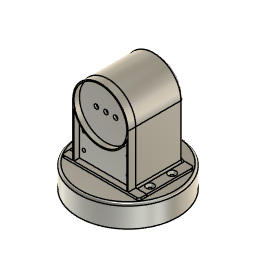
TRARM02_Link1 (Autodesk Fusion 360 design; units mm, degrees)
Autodesk Fusion 360 part; units mm, degrees
sketch "스케치1" plane through (0, 0, 0) normal (0, 0, 1) x (1, 0, 0) in component "TRARM02_Link1A_R90x20 v1"
  circle A0 centre (0, 0) radius 45
  dimension "d1" = 90
  constraint coincident A0.centre origin
  measures "d1" diameter of A0
extrude "돌출1" add sketch "스케치1" along normal blind 2 makes body 1 in component "TRARM02_Link1A_R90x20 v1"
sketch "스케치2" plane through (0, 0, 2) normal (0, 0, 1) x (-1, 0, 0) in component "TRARM02_Link1A_R90x20 v1"
  circle A0 centre (0, 0) radius 45
  circle A1 centre (0, 0) radius 43
  dimension "d4" = 86
  dimension "d5" = 90
  constraint coincident A0.centre A1.centre
  measures "d4" diameter of A1
  measures "d5" diameter of A0
extrude "돌출2" add sketch "스케치2" along normal blind 18 bodies 1 in component "TRARM02_Link1A_R90x20 v1"
fillet "필렛1" radius 2 1 edges at (-41.9547, -16.2727, 0) on bodies 1 in component "TRARM02_Link1A_R90x20 v1"
sketch "스케치4" plane through (0, 0, 2) normal (0, 0, 1) x (-1, 0, 0) in component "TRARM02_Link1A_R90x20 v1"
  circle A0 centre (0, 0) radius 43
  line L0 (-30, -13) -> (-40.9878, -13)
  line L1 (-30, -7) -> (-42.4264, -7)
  line L2 (-30, 7) -> (-42.4264, 7)
  line L3 (-30, 13) -> (-40.9878, 13)
  line L4 (30, -13) -> (40.9878, -13)
  line L5 (30, -7) -> (42.4264, -7)
  line L6 (30, 7) -> (42.4264, 7)
  line L7 (30, 13) -> (40.9878, 13)
  arc A1 (30, 13) -> (30, 7) centre (30, 10) ccw
  arc A2 (30, -7) -> (30, -13) centre (30, -10) ccw
  arc A3 (-30, -13) -> (-30, -7) centre (-30, -10) ccw
  arc A4 (-30, 7) -> (-30, 13) centre (-30, 10) ccw
  dimension "d32" = 6
  dimension "d33" = 60
  dimension "d34" = 20
  dimension "d35" = 10
  dimension "d36" = 30
  dimension "d46" = 6
  dimension "d47" = 6
  constraint equal A2 A3
  constraint equal A1 A2
  constraint equal A1 A4
  constraint horizontal A2.centre A3.centre
  constraint horizontal A1.centre A4.centre
  constraint vertical A2.centre A1.centre
  constraint vertical A3.centre A4.centre
  constraint coincident A0 L0.end
  constraint coincident A0 L1.end
  constraint horizontal L0
  constraint horizontal L1
  constraint coincident A0 L2.end
  constraint coincident A0 L3.end
  constraint horizontal L2
  constraint horizontal L3
  constraint coincident A0 L4.end
  constraint coincident A0 L5.end
  constraint horizontal L4
  constraint horizontal L5
  constraint coincident A0 L6.end
  constraint coincident A0 L7.end
  constraint horizontal L6
  constraint horizontal L7
  constraint vertical L6.start L7.start
  constraint vertical L5.start L7.start
  constraint vertical L4.start L5.start
  constraint vertical L0.start L1.start
  constraint vertical L1.start L2.start
  constraint vertical L2.start L3.start
  measures "d32" diameter of A3
  measures "d33" distance of A2.centre A3.centre
  measures "d34" distance of A2.centre A1.centre
  measures "d35" vertical distance of A0.centre A1.centre
  measures "d36" horizontal distance of A0.centre A2.centre
  measures "d46" distance of L4 L5
  measures "d47" distance of L0 L1
extrude "돌출7" add sketch "스케치4" along normal blind 5 contours A0 L6 L7 A1 | A0 L4 L5 A2 | A0 L2 L3 A4 | A0 L0 L1 A3 bodies 1 in component "TRARM02_Link1A_R90x20 v1"
sketch "스케치7" plane through (0, 0, 0) normal (0, 0, -1) x (1, 0, 0) in component "TRARM02_Link1A_R90x20 v1"
  arc A0 (-30, -13) -> (-30, -7) centre (-30, -10) ccw construction
  arc A1 (-30, 7) -> (-30, 13) centre (-30, 10) ccw construction
  arc A2 (30, 13) -> (30, 7) centre (30, 10) ccw construction
  arc A3 (30, -7) -> (30, -13) centre (30, -10) ccw construction
  circle A4 centre (-30, 10) radius 1.45
  circle A5 centre (-30, -10) radius 1.45
  circle A6 centre (30, -10) radius 1.45
  circle A7 centre (30, 10) radius 1.45
  dimension "d42" = 2.9
  constraint concentric A1 A4
  constraint concentric A0 A5
  constraint concentric A3 A6
  constraint concentric A2 A7
  constraint equal A6 A7
  constraint equal A5 A6
  constraint equal A4 A5
  measures "d42" diameter of A7
extrude "돌출8" cut sketch "스케치7" against normal blind 5 bodies 1 in component "TRARM02_Link1A_R90x20 v1"
fillet "필렛2" radius 1 12 edges at (-35.4939, -13, 7) (-27, -10, 7) (-36.2132, -7, 7) (-36.2132, 7, 7) (-27, 10, 7) (-35.4939, 13, 7) (35.4939, 13, 7) (27, 10, 7) (36.2132, 7, 7) (36.2132, -7, 7) (27, -10, 7) (35.4939, -13, 7) on bodies 1 in component "TRARM02_Link1A_R90x20 v1"
sketch "스케치9" plane through (0, 0, 2) normal (0, 0, 1) x (-1, 0, 0) in component "TRARM02_Link1A_R90x20 v1"
  circle A0 centre (0, 0) radius 15
  dimension "d50" = 30
  constraint coincident A0.centre origin
  measures "d50" diameter of A0
extrude "돌출9" add sketch "스케치9" along normal blind 1 bodies 1 in component "TRARM02_Link1A_R90x20 v1"
sketch "스케치10" plane through (0, 0, 3) normal (0, 0, 1) x (-1, 0, 0) in component "TRARM02_Link1A_R90x20 v1"
  circle A0 centre (0, 0) radius 2
  circle A1 centre (-8.7, 0) radius 2
  circle A2 centre (8.7, 0) radius 2
  dimension "d53" = 8.7
  dimension "d54" = 8.7
  dimension "d55" = 4
  constraint coincident A0.centre origin
  constraint equal A0 A2
  constraint equal A1 A2
  constraint horizontal A0.centre A1.centre
  constraint horizontal A0.centre A2.centre
  measures "d53" distance of A0.centre A1.centre
  measures "d54" distance of A0.centre A2.centre
  measures "d55" diameter of A1
extrude "돌출10" cut sketch "스케치10" against normal blind 3 bodies 1 in component "TRARM02_Link1A_R90x20 v1"
sketch "스케치11" plane through (0, 0, 0) normal (0, 0, -1) x (1, 0, 0) in component "TRARM02_Link1A_R90x20 v1"
  line L0 (21, 5) -> (21, -5)
  line L1 (16, -5) -> (16, 5)
  line L2 (-16, 5) -> (-16, -5)
  line L3 (-21, -5) -> (-21, 5)
  arc A0 (-16, 5) -> (-21, 5) centre (-18.5, 5) ccw
  arc A1 (-21, -5) -> (-16, -5) centre (-18.5, -5) ccw
  arc A2 (16, -5) -> (21, -5) centre (18.5, -5) ccw
  arc A3 (21, 5) -> (16, 5) centre (18.5, 5) ccw
  dimension "d58" = 5
  dimension "d60" = 10
  dimension "d61" = 16
  dimension "d62" = 5
  dimension "d63" = 16
  dimension "d64" = 2.5
  dimension "d65" = 5
  constraint vertical L0
  constraint vertical L1
  constraint vertical L2
  constraint vertical L3
  constraint equal L0 L2
  constraint horizontal L1.start L2.end
  constraint equal A2 A3
  constraint equal A0 A1
  constraint equal A0 A2
  constraint horizontal L3.end L2.start
  constraint horizontal L1.end L3.end
  constraint horizontal L1.end L0.start
  constraint equal L2 L3
  measures "d58" distance of L0.end L1.start
  measures "d60" distance of L0.start L0.end
  measures "d61" horizontal distance of origin L1.start
  measures "d62" vertical distance of origin L1.start
  measures "d63" horizontal distance of origin L2.end
  measures "d64" radius of A2
  measures "d65" distance of L2 L3
extrude "돌출11" cut sketch "스케치11" against normal blind 2 bodies 1 in component "TRARM02_Link1A_R90x20 v1"
move_body "이동1" bodies 1 to x (1, 0, 0) y (0, -1, 0) z (0, 0, -1) at (0, 0, 0) in component "TRARM02_Link1A_R90x20 v1"
move_body "이동2" bodies 1 to x (1, 0, 0) y (0, 1, 0) z (0, 0, 1) at (0, 0, 20) in component "TRARM02_Link1A_R90x20 v1"
move_body "이동3" bodies 1 to x (0, 1, 0) y (-1, 0, 0) z (0, 0, 1) at (0, 0, 0) in component "TRARM02_Link1A_R90x20 v1"
move_body "이동4" bodies 1 to x (0, 1, 0) y (-1, 0, 0) z (0, 0, 1) at (0, 0, 0) in component "TRARM02_Link1A_R90x20 v1"
sketch "스케치1 (2)" plane through (0, 0, 0) normal (0, 0, 1) x (1, 0, 0) in component "TRARM02_Link1B_50x50x43 v1"
  line L0 (25, 50) -> (25, 2)
  line L1 (-25, 50) -> (-25, 2)
  arc A0 (25, 50) -> (-25, 50) centre (0, 50) ccw
  line L2 (-35, 0) -> (-35, 2)
  line L3 (-35, 2) -> (-25, 2)
  line L4 (35, 0) -> (35, 2)
  line L5 (35, 2) -> (25, 2)
  line L6 (-35, 0) -> (35, 0)
  dimension "d222" = 25
  dimension "d223" = 50
  dimension "d224" = 2
  dimension "d225" = 10
  constraint vertical origin A0.centre
  constraint vertical L0
  constraint tangent L1 A0
  constraint parallel L0 L1
  constraint vertical L2
  constraint horizontal L3
  constraint vertical L4
  constraint horizontal L5
  constraint perpendicular L2 L6
  constraint equal L2 L4
  constraint equal L3 L5
  constraint tangent L0 A0
  constraint coincident origin L6
  measures "d222" radius of A0
  measures "d223" distance of origin A0.centre
  measures "d224" distance of L4.start L4.end
  measures "d225" distance of L4.end L0.end
extrude "돌출1'" add sketch "스케치1 (2)" along normal blind 43 separate body makes body 2 in component "TRARM02_Link1B_50x50x43 v1"
sketch "스케치27" plane through (0, 0, 43) normal (0, 0, 1) x (-1, 0, 0) in component "TRARM02_Link1B_50x50x43 v1"
  line L0 (35, 0) -> (-35, 0)
  line L1 (24, -2) -> (-24, -2)
  line L2 (-20, -22) -> (-24, -22)
  line L3 (-20, -28) -> (-24, -28)
  line L4 (-20, -13) -> (-24, -13)
  line L5 (-20, -7) -> (-24, -7)
  line L6 (20, -13) -> (24, -13)
  line L7 (20, -7) -> (24, -7)
  line L8 (20, -22) -> (24, -22)
  line L9 (20, -28) -> (24, -28)
  arc A0 (20.0014, -22) -> (20, -28) centre (20, -25) ccw
  line L10 (24, -50) -> (24, -28)
  line L11 (24, -22) -> (24, -13)
  line L12 (24, -7) -> (24, -2)
  arc A1 (20, -7) -> (20, -13) centre (20, -10) ccw
  arc A2 (-20, -13) -> (-20, -7) centre (-20, -10) ccw
  line L13 (-24, -7) -> (-24, -2)
  arc A3 (-20, -28) -> (-20.0014, -22) centre (-20, -25) ccw
  line L14 (-24, -50) -> (-24, -28)
  line L15 (-24, -22) -> (-24, -13)
  line L16 (-3, -70) -> (-3, -73.8118)
  line L17 (3, -70) -> (3, -73.8118)
  arc A4 (3, -70) -> (-3, -70) centre (0, -70) ccw
  arc A5 (-24, -50) -> (-3, -73.8118) centre (0, -50) ccw
  arc A6 (3, -73.8118) -> (24, -50) centre (0, -50) ccw
  dimension "d246" = 48
  dimension "d247" = 50
  dimension "d248" = 2
  dimension "d251" = 6
  dimension "d252" = 20
  dimension "d253" = 25
  dimension "d254" = 15
  dimension "d255" = 20
  dimension "d279" = 6
  dimension "d280" = 20
  constraint parallel L0 L1
  constraint coincident L1 L13.end
  constraint vertical L10
  constraint vertical L14
  constraint coincident L1.end L13.end
  constraint tangent L14 A5
  constraint tangent L10 A5
  constraint vertical origin A5.centre
  constraint equal A0 A1
  constraint equal A0 A3
  constraint equal A2 A3
  constraint horizontal A2.centre A1.centre
  constraint horizontal A0.centre A3.centre
  constraint vertical A3.centre A2.centre
  constraint vertical A0.centre A1.centre
  constraint coincident L2.start A3
  constraint coincident L2.end L14
  constraint perpendicular L2 L14
  constraint perpendicular L3 L14
  constraint perpendicular L4 L14
  constraint coincident L5.end L14
  constraint perpendicular L5 L14
  constraint coincident L6.end L10
  constraint perpendicular L6 L10
  constraint coincident L7.end L10
  constraint perpendicular L7 L10
  constraint coincident L8.start A0
  constraint coincident L8.end L10
  constraint perpendicular L8 L10
  constraint perpendicular L9 L10
  constraint coincident L8 A0.start
  constraint collinear L10 L11
  constraint collinear L11 L12
  constraint collinear L13 L14
  constraint coincident L2 A3.end
  constraint collinear L14 L15
  constraint equal L2 L3
  constraint equal L2 L4
  constraint equal L4 L5
  constraint equal L5 L7
  constraint equal L6 L7
  constraint equal L6 L8
  constraint equal L8 L9
  constraint vertical A5.centre A4.centre
  constraint vertical L16
  constraint coincident L17.end A5
  constraint parallel L16 L17
  constraint concentric A5 A6
  constraint horizontal A4.centre L17.start
  constraint horizontal L16.start L17.start
  measures "d246" diameter of A5
  measures "d247" distance of origin A5.centre
  measures "d248" distance of origin L1
  measures "d251" diameter of A3
  measures "d252" horizontal distance of A5.centre A3.centre
  measures "d253" vertical distance of A5.centre A3.centre
  measures "d254" vertical distance of A3.centre A2.centre
  measures "d255" horizontal distance of A5.centre A0.centre
  measures "d279" diameter of A4
  measures "d280" distance of A5.centre A4.centre
extrude "돌출32" cut sketch "스케치27" against normal blind 41 bodies 2 in component "TRARM02_Link1B_50x50x43 v1"
sketch "스케치28" plane through (0, 0, 43) normal (0, 0, 1) x (-1, 0, 0) in component "TRARM02_Link1B_50x50x43 v1"
  circle A0 centre (-20, -25) radius 1.45
  circle A1 centre (-20, -10) radius 1.45
  circle A2 centre (20, -10) radius 1.45
  circle A3 centre (20, -25) radius 1.45
  arc A4 (-20, -28) -> (-20.0014, -22) centre (-20, -25) ccw
  arc A5 (-20, -13) -> (-20, -7) centre (-20, -10) ccw
  arc A6 (20, -7) -> (20, -13) centre (20, -10) ccw
  arc A7 (20.0014, -22) -> (20, -28) centre (20, -25) ccw
  circle A8 centre (0, -70) radius 1.45
  arc A9 (3, -70) -> (-3, -70) centre (0, -70) ccw
  dimension "d258" = 2.9
  constraint equal A0 A3
  constraint equal A0 A1
  constraint concentric A0 A4
  constraint concentric A1 A5
  constraint concentric A2 A6
  constraint concentric A3 A7
  constraint equal A0 A2
  constraint concentric A8 A9
  constraint equal A0 A8
  measures "d258" diameter of A0
extrude "돌출33" cut sketch "스케치28" against normal blind 5 bodies 2 in component "TRARM02_Link1B_50x50x43 v1"
fillet "필렛6" radius 2 3 edges at (-25, 26, 0) (0, 75, 0) (25, 26, 0) on bodies 2 in component "TRARM02_Link1B_50x50x43 v1"
fillet "필렛6" radius 2 2 edges at (35, 1, 0) (-35, 1, 0) on bodies 2 in component "TRARM02_Link1B_50x50x43 v1"
sketch "스케치29" plane through (0, 2, 0) normal (0, 1, 0) x (-1, 0, 0) in component "TRARM02_Link1B_50x50x43 v1"
  circle A0 centre (30, 15) radius 1.5
  circle A1 centre (30, 35) radius 1.5
  line L0 (25, 43) -> (35, 43)
  circle A2 centre (-30, 15) radius 1.5
  circle A3 centre (-30, 35) radius 1.5
  point P0 (-35, 43)
  dimension "d265" = 3
  dimension "d266" = 5
  dimension "d268" = 15
  dimension "d269" = 20
  dimension "d281" = 60
  constraint equal A2 A3
  constraint equal A0 A2
  constraint equal A0 A1
  constraint vertical A2.centre A3.centre
  constraint vertical A0.centre A1.centre
  constraint horizontal A0.centre A2.centre
  constraint horizontal A1.centre A3.centre
  measures "d265" diameter of A2
  measures "d266" horizontal distance of A1.centre L0.end
  measures "d268" vertical distance of origin A2.centre
  measures "d269" distance of A2.centre A3.centre
  measures "d281" distance of A1.centre A3.centre
extrude "돌출34" cut sketch "스케치29" against normal blind 2 bodies 2 in component "TRARM02_Link1B_50x50x43 v1"
chamfer "챔퍼6" distance 2 angle 45 4 edges at (31.3985, 2, 15.5424) (31.3985, 2, 35.5424) (-28.6015, 2, 35.5424) (-28.6015, 2, 15.5424) on bodies 2 in component "TRARM02_Link1B_50x50x43 v1"
fillet "필렛7" radius 1.4 4 edges at (24.4142, 2, 0.5858) (25, 2, 22.5) (-24.4142, 2, 0.5858) (-25, 2, 22.5) on bodies 2 in component "TRARM02_Link1B_50x50x43 v1"
sketch "스케치30" plane through (0, 0, 0) normal (0, -1, 0) x (1, 0, 0) in component "TRARM02_Link1B_50x50x43 v1"
  circle A0 centre (0, 25) radius 15
  line L0 (21, 30) -> (21, 20)
  line L1 (16, 20) -> (16, 30)
  arc A1 (21, 30) -> (16, 30) centre (18.5, 30) ccw
  arc A2 (16, 20) -> (21, 20) centre (18.5, 20) ccw
  line L2 (-16, 30) -> (-16, 20)
  line L3 (-21, 20) -> (-21, 30)
  arc A3 (-16, 30) -> (-21, 30) centre (-18.5, 30) ccw
  arc A4 (-21, 20) -> (-16, 20) centre (-18.5, 20) ccw
  dimension "d275" = 30
  dimension "d276" = 25
  dimension "d282" = 10
  dimension "d283" = 5
  dimension "d284" = 16
  dimension "d285" = 20
  dimension "d286" = 2.5
  dimension "d287" = 16
  dimension "d288" = 5
  dimension "d289" = 10
  dimension "d290" = 20
  dimension "d291" = 2.5
  constraint vertical origin A0.centre
  constraint vertical L0
  constraint vertical L1
  constraint equal A1 A2
  constraint equal L0 L1
  constraint horizontal L1.end L0.start
  constraint vertical L2
  constraint vertical L3
  constraint equal A3 A4
  constraint equal L2 L3
  constraint horizontal L2.end A4.centre
  constraint horizontal L2.end L3.start
  measures "d275" diameter of A0
  measures "d276" distance of origin A0.centre
  measures "d282" distance of L0.start L0.end
  measures "d283" distance of L0.end L1.start
  measures "d284" horizontal distance of origin L1.start
  measures "d285" vertical distance of origin L1.start
  measures "d286" radius of A2
  measures "d287" horizontal distance of origin L2.end
  measures "d288" distance of L3.end L2.start
  measures "d289" distance of L3.end L3.start
  measures "d290" vertical distance of origin L2.end
  measures "d291" radius of A4
extrude "돌출35" cut sketch "스케치30" against normal blind 2 bodies 2 in component "TRARM02_Link1B_50x50x43 v1"
sketch "스케치1 (3)" plane through (0, 0, 0) normal (0, 0, 1) x (1, 0, 0) in component "TRARM02_Link1C_50x50x7 v1"
  line L0 (25, 50) -> (25, 2)
  line L1 (-25, 50) -> (-25, 2)
  arc A0 (25, 50) -> (-25, 50) centre (0, 50) ccw
  line L2 (-35, 0) -> (-35, 2)
  line L3 (-35, 2) -> (-25, 2)
  line L4 (35, 0) -> (35, 2)
  line L5 (35, 2) -> (25, 2)
  line L6 (-35, 0) -> (35, 0)
  dimension "d222_1" = 25
  dimension "d223_1" = 50
  dimension "d224_1" = 2
  dimension "d225_1" = 10
  constraint vertical origin A0.centre
  constraint vertical L0
  constraint tangent L1 A0
  constraint parallel L0 L1
  constraint vertical L2
  constraint horizontal L3
  constraint vertical L4
  constraint horizontal L5
  constraint perpendicular L2 L6
  constraint equal L2 L4
  constraint equal L3 L5
  constraint tangent L0 A0
  constraint coincident origin L6
  measures "d222_1" radius of A0
  measures "d223_1" distance of origin A0.centre
  measures "d224_1" distance of L4.start L4.end
  measures "d225_1" distance of L4.end L0.end
extrude "돌출1''" add sketch "스케치1 (3)" along normal blind 7 separate body makes body 3 in component "TRARM02_Link1C_50x50x7 v1"
sketch "스케치24" plane through (0, 0, 7) normal (0, 0, 1) x (-1, 0, 0) in component "TRARM02_Link1C_50x50x7 v1"
  circle A0 centre (0, -50) radius 24
  circle A1 centre (0, -50) radius 25
  line L0 (35, 0) -> (-35, 0)
  line L1 (24, -2) -> (-24, -2)
  line L2 (-24, -2) -> (-24, -43)
  line L3 (24, -2) -> (24, -43)
  line L4 (-25, -2) -> (-25, -50)
  line L5 (25, -50) -> (25, -2)
  point P0 (-25, -50)
  dimension "d226" = 48
  dimension "d227" = 1
  dimension "d228" = 1
  constraint concentric A0 A1
  constraint coincident A1 P0
  constraint parallel L0 L1
  constraint coincident A1 L2.end
  constraint perpendicular L1 L2
  constraint coincident A1 L3.end
  constraint perpendicular L1 L3
  constraint horizontal L1.end L4.start
  measures "d226" diameter of A0
  measures "d227" distance of L2 L4
  measures "d228" distance of L3 L5
extrude "돌출28" cut sketch "스케치24" against normal blind 5 contours A0 | A1 L1 L2 L3 bodies 3 in component "TRARM02_Link1C_50x50x7 v1"
sketch "스케치25" plane through (0, 0, 2) normal (0, 0, 1) x (-1, 0, 0) in component "TRARM02_Link1C_50x50x7 v1"
  circle A0 centre (0, -50) radius 2
  circle A1 centre (-8.7, -50) radius 2
  circle A2 centre (8.7, -50) radius 2
  dimension "d231" = 4
  dimension "d232" = 50
  dimension "d233" = 8.7
  dimension "d234" = 8.7
  constraint equal A0 A2
  constraint equal A0 A1
  constraint horizontal A0.centre A1.centre
  constraint horizontal A0.centre A2.centre
  constraint vertical origin A0.centre
  measures "d231" diameter of A1
  measures "d232" distance of origin A0.centre
  measures "d233" distance of A0.centre A1.centre
  measures "d234" distance of A0.centre A2.centre
extrude "돌출29" cut sketch "스케치25" against normal blind 2 bodies 3 in component "TRARM02_Link1C_50x50x7 v1"
sketch "스케치26" plane through (0, 0, 2) normal (0, 0, 1) x (-1, 0, 0) in component "TRARM02_Link1C_50x50x7 v1"
  circle A0 centre (-20, -25) radius 1.5
  circle A1 centre (20, -25) radius 1.5
  circle A2 centre (20, -10) radius 1.5
  circle A3 centre (-20, -10) radius 1.5
  circle A4 centre (0, -50) radius 2
  circle A5 centre (0, -70) radius 1.5
  dimension "d237" = 25
  dimension "d238" = 3
  dimension "d239" = 20
  dimension "d240" = 20
  dimension "d241" = 15
  dimension "d246_1" = 20
  constraint equal A0 A1
  constraint horizontal A0.centre A1.centre
  constraint equal A0 A3
  constraint equal A1 A2
  constraint vertical A0.centre A3.centre
  constraint vertical A1.centre A2.centre
  constraint horizontal A2.centre A3.centre
  constraint equal A3 A5
  measures "d237" vertical distance of A0.centre A4.centre
  measures "d238" diameter of A3
  measures "d239" horizontal distance of A0.centre A4.centre
  measures "d240" horizontal distance of A1.centre A4.centre
  measures "d241" distance of A0.centre A3.centre
  measures "d246_1" distance of A4.centre A5.centre
extrude "돌출30" cut sketch "스케치26" against normal blind 2 contours A0 | A1 | A2 | A3 | A5 bodies 3 in component "TRARM02_Link1C_50x50x7 v1"
fillet "필렛5" radius 2 2 edges at (-35, 1, 7) (35, 1, 7) on bodies 3 in component "TRARM02_Link1C_50x50x7 v1"
component "TRARM02_Link1A_R90x20 v1" placed x (1, 0, 0) y (0, 1, 0) z (0, 0, 1) at (0, 0, 0)
component "TRARM02_Link1B_50x50x43 v1" placed x (1, 0, 0) y (0, 0, 1) z (0, -1, 0) at (0, 25, 20)
component "TRARM02_Link1C_50x50x7 v1" placed x (1, 0, 0) y (0, 0, 1) z (0, -1, 0) at (0, -18, 20)
